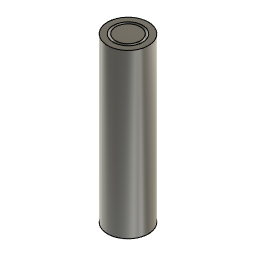
röratest (Autodesk Fusion 360 design; units mm, degrees)
Autodesk Fusion 360 part; units mm, degrees
sketch "Sketch1" plane through (0, 0, 0) normal (0, 0, 1) x (1, 0, 0)
  circle A0 centre (0, 0) radius 2.5
  circle A1 centre (0, 0) radius 1.8
  circle A2 centre (0, 0) radius 1.5
  dimension "d1" = 5
  dimension "d2" = 3.6
  dimension "d3" = 3
  constraint coincident A0.centre A1.centre
  constraint concentric A0 A1
  constraint concentric A0 A2
  measures "d1" diameter of A0
  measures "d2" diameter of A1
  measures "d3" diameter of A2
extrude "Extrude1" add sketch "Sketch1" along normal blind 20 makes body 1 at (2.4969, -0.1246, 13.3333) makes body 2 at (1.4981, -0.0748, 13.3333)
